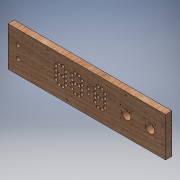
# Autodesk Inventor part: licht_200_top_b
Saved by Autodesk Inventor 2016 SP2 (Build 200236200, 236)
## iProperties
Created: 2018-01-11
Part Number: licht_200_top_b
Material: Spanplatte
Document SubType Name: Blech
Designer: schueler
Density: 1 g/cm^3
Sheet Metal Rule: Standard_mm
Appearance: Birke - natur- poliert
Mass: 590.035 g
Surface Area: 1129.46 cm^2
Volume: 590.035 cm^3
Author: schueler
Autodesk Inventor part; units mm, degrees
ref_plane "YZ Plane" through (0, 0, 0) normal (1, 0, 0) x (0, 1, 0)
ref_plane "XZ Plane" through (0, 0, 0) normal (0, 1, 0) x (-1, 0, 0)
ref_plane "XY Plane" through (0, 0, 0) normal (0, 0, 1) x (1, 0, 0)
sketch "Skizze1" plane through (0, 0, 0) normal (0, 1, 0) x (-1, 0, 0)
  line L0 (0, 0) -> (400, 0)
  line L1 (400, -100) -> (0, -100)
  line L2 (0, -100) -> (0, 0)
  line L3 (100, 0) -> (100, -100) construction
  line L4 (0, -92) -> (400, -92) construction
  circle A0 centre (100, -8) radius 1.5
  line L5 (8, 0) -> (8, -100) construction
  circle A1 centre (8, -30) radius 1.5
  circle A2 centre (8, -70) radius 1.5
  line L6 (400, -8) -> (0, -8) construction
  circle A3 centre (250, -92) radius 1.5
  line L7 (300, 0) -> (300, -100) construction
  circle A4 centre (300, -8) radius 1.5
  line L8 (400, -100) -> (400, 0)
  line L9 (250, -8) -> (250, -92) construction
  point P0 (100, -92)
  point P1 (100, -8)
  point P2 (300, -92)
  dimension "d2" = 400
  dimension "d7" = 100
  dimension "d16" = 3
  dimension "d19" = 8
  dimension "d23" = 3
  dimension "d24" = 3
  dimension "d46" = 30
  dimension "d47" = 30
  dimension "d57" = 8
  dimension "d58" = 3
  dimension "d63" = 200
  dimension "d69" = 3
  dimension "d116" = 250
  dimension "d127" = 100
  dimension "d128" = 8
  constraints: 22 point on line, 21 end point, 5 centre point, 5 perpendicular, 1 coincident, 1 horizontal, 1 parallel, 1 vertical
  measures "d2" distance of L1.start L1.end
  measures "d7" distance of L0.start L3.start
  measures "d16" diameter of A0
  measures "d19" distance of L0.start L5.start
  measures "d23" diameter of A1
  measures "d24" diameter of A2
  measures "d46" distance from line of L0 A1.centre
  measures "d47" distance from line of L1 A2.centre
  measures "d57" distance between parallel lines of L0 L6
  measures "d58" diameter of A3
  measures "d63" distance between parallel lines of L3 L7
  measures "d69" diameter of A4
  measures "d116" distance from line of L2 L9.start
  measures "d127" distance between parallel lines of L0 L1
  measures "d128" distance between parallel lines of L1 L4
extrude "Extrusion9" add sketch "Skizze1" along normal blind 16
sketch "Skizze6" plane through (0, 0, 0) normal (0, -1, 0) x (1, 0, 0)
  line L0 (-400, -100) -> (0, -100) construction
  line L1 (0, -100) -> (0, 0) construction
  line L2 (0, 0) -> (-400, 0) construction
  line L3 (-400, 0) -> (-400, -100) construction
  line L4 (0, -50) -> (-400, -50) construction
  line L5 (-400, 0) -> (-400, -100) construction
  line L6 (0, 0) -> (-400, 0) construction
  line L7 (-400, -100) -> (0, -100) construction
  line L8 (-254, 0) -> (-254, -100) construction
  line L9 (-261.5, 0) -> (-261.5, -100) construction
  line L10 (-271.5, 0) -> (-271.5, -100) construction
  line L11 (-279, 0) -> (-279, -100) construction
  line L12 (-238, 0) -> (-238, -100) construction
  line L13 (-230.5, 0) -> (-230.5, -100) construction
  line L14 (-220.5, 0) -> (-220.5, -100) construction
  line L15 (-213, 0) -> (-213, -102.7121) construction
  line L16 (-179, 0) -> (-179, -100) construction
  line L17 (-171.5, 0) -> (-171.5, -100) construction
  line L18 (-161.5, 0) -> (-161.5, -100) construction
  line L19 (-154, 0) -> (-154, -100) construction
  line L20 (-279, -41.5) -> (-154, -41.5) construction
  line L21 (-154, -31.5) -> (-279, -31.5) construction
  line L22 (-279, -24) -> (-154, -24) construction
  line L23 (-279, -51.5) -> (-154, -51.5) construction
  line L24 (-154, -61.5) -> (-279, -61.5) construction
  line L25 (-279, -69) -> (-154, -69) construction
  line L26 (-250, 0) -> (-250, -100) construction
  line L27 (-196, -61.5) -> (-196, -41.5) construction
  point P0 (-271.5, -69)
  point P1 (-261.5, -69)
  point P2 (-254, -61.5)
  point P3 (-254, -51.5)
  point P4 (-271.5, -24)
  point P5 (-261.5, -24)
  point P6 (-254, -31.5)
  point P7 (-254, -41.5)
  point P8 (-238, -41.5)
  point P9 (-238, -31.5)
  point P10 (-230.5, -24)
  point P11 (-220.5, -24)
  point P12 (-213, -31.5)
  point P13 (-213, -41.5)
  point P14 (-238, -51.5)
  point P15 (-238, -61.5)
  point P16 (-230.5, -69)
  point P17 (-220.5, -69)
  point P18 (-213, -61.5)
  point P19 (-213, -51.5)
  point P20 (-171.5, -24)
  point P21 (-161.5, -24)
  point P22 (-179, -31.5)
  point P23 (-179, -41.5)
  point P24 (-161.5, -69)
  point P25 (-171.5, -69)
  point P26 (-179, -61.5)
  point P27 (-179, -51.5)
  point P28 (-375, -35)
  point P29 (-375, -65)
  point P30 (-196, -52)
  point P31 (-196, -41)
  point P32 (-271.5, -46.5)
  point P33 (-261.5, -46.5)
  point P34 (-230.5, -46.5)
  point P35 (-220.5, -46.5)
  point P36 (-171.5, -46.5)
  point P37 (-161.5, -46.5)
  dimension "d137" = 7.5
  dimension "d139" = 7.5
  dimension "d141" = 7.5
  dimension "d143" = 7.5
  dimension "d145" = 7.5
  dimension "d147" = 7.5
  dimension "d149" = 10
  dimension "d150" = 7.5
  dimension "d152" = 10
  dimension "d153" = 7.5
  dimension "d201" = 17
  dimension "d215" = 25
  dimension "d216" = 66
  dimension "d217" = 25
  dimension "d218" = 25
  dimension "d220" = 17
  dimension "d221" = 154
  dimension "d222" = 45
  dimension "d223" = 24
  dimension "d224" = 15
  dimension "d225" = 15
  dimension "d226" = 25
  dimension "d228" = 11
  dimension "d229" = 10
  dimension "d230" = 5
  dimension "d232" = 48
  constraints: 78 point on line, 50 end point, 12 perpendicular, 8 coincident, 8 parallel, 5 horizontal alignment, 3 vertical, 2 midpoint, 1 horizontal, 1 vertical alignment, 27 other
  measures "d137" distance between parallel lines of L12 L13
  measures "d139" distance between parallel lines of L15 L14
  measures "d141" distance between parallel lines of L9 L8
  measures "d143" distance between parallel lines of L10 L11
  measures "d145" distance between parallel lines of L17 L16
  measures "d147" distance between parallel lines of L19 L18
  measures "d149" distance between parallel lines of L20 L21
  measures "d150" distance between parallel lines of L21 L22
  measures "d152" distance between parallel lines of L23 L24
  measures "d153" distance between parallel lines of L24 L25
  measures "d201" distance between parallel lines of L15 L27
  measures "d215" distance between parallel lines of L19 L16
  measures "d216" distance between parallel lines of L11 L15
  measures "d217" distance between parallel lines of L11 L8
  measures "d218" distance between parallel lines of L12 L15
  measures "d220" distance between parallel lines of L16 L27
  measures "d221" distance between parallel lines of L19 L1
  measures "d222" distance between parallel lines of L25 L22
  measures "d223" distance between parallel lines of L2 L22
  measures "d224" distance from line of point (-375, -35) L4
  measures "d225" distance from line of L4 point (-375, -65)
  measures "d226" distance from line of L3 point (-375, -65)
  measures "d228" distance of point (-196, -41) point (-196, -52)
  measures "d229" distance of L23.start point (-279, -41.5)
  measures "d230" distance from line of point (-271.5, -46.5) L20
hole "Bohrung5" at (-271.5, 0, -69) at (-261.5, 0, -69) at (-254, 0, -61.5) at (-254, 0, -51.5) at (-279, 0, -51.5) at (-279, 0, -61.5) at (-279, 0, -41.5) at (-279, 0, -31.5) at (-271.5, 0, -24) at (-261.5, 0, -24) at (-254, 0, -31.5) at (-254, 0, -41.5) at (-238, 0, -41.5) at (-238, 0, -31.5) at (-230.5, 0, -24) at (-220.5, 0, -24) at (-213, 0, -31.5) at (-213, 0, -41.5) at (-238, 0, -51.5) at (-238, 0, -61.5) at (-230.5, 0, -69) at (-220.5, 0, -69) at (-213, 0, -61.5) at (-213, 0, -51.5) at (-171.5, 0, -24) at (-161.5, 0, -24) at (-179, 0, -31.5) at (-179, 0, -41.5) at (-154, 0, -51.5) at (-154, 0, -61.5) at (-161.5, 0, -69) at (-171.5, 0, -69) at (-179, 0, -61.5) at (-179, 0, -51.5) at (-154, 0, -41.5) at (-154, 0, -31.5) at (-196, 0, -41) at (-196, 0, -52) at (-271.5, 0, -46.5) at (-261.5, 0, -46.5) at (-230.5, 0, -46.5) at (-220.5, 0, -46.5) at (-171.5, 0, -46.5) at (-161.5, 0, -46.5) direction (0, 1, 0) diameter 6 depth 30 tip angle 118 counterbore diameter 8 counterbore depth 12
hole "Bohrung6" at (-375, 0, -35) at (-375, 0, -65) direction (0, 1, 0) diameter 7 depth 30 tip angle 118 counterbore diameter 10 counterbore depth 12
sketch "Skizze7" plane through (0, 16, 0) normal (0, 1, 0) x (1, 0, 0)
  circle A0 centre (-250, 92) radius 1.5 projected
  circle A1 centre (-300, 8) radius 1.5 projected
  circle A2 centre (-8, 70) radius 1.5 projected
  circle A3 centre (-8, 30) radius 1.5 projected
  circle A4 centre (-100, 8) radius 1.5 projected
  line L0 (0, 0) -> (-400, 0) construction
  line L1 (-400, 0) -> (-400, 100) construction
  line L2 (-400, 100) -> (0, 100) construction
  line L3 (0, 100) -> (0, 0) construction
  line L4 (-40, 50) -> (0, 50) construction
  line L5 (0, 0) -> (0, 100) construction
  line L6 (-25.4, 35.4) -> (-54.6, 35.4) construction
  line L7 (-54.6, 35.4) -> (-54.6, 64.6) construction
  line L8 (-54.6, 64.6) -> (-25.4, 64.6) construction
  line L9 (-25.4, 64.6) -> (-25.4, 35.4) construction
  line L10 (-40, 50) -> (-40, 100) construction
  circle A5 centre (-40, 50) radius 25.4 construction
  line L11 (-100, 0) -> (-100, 100) construction
  line L12 (-85.4, 35.4) -> (-114.6, 35.4) construction
  line L13 (-114.6, 35.4) -> (-114.6, 64.6) construction
  line L14 (-114.6, 64.6) -> (-85.4, 64.6) construction
  line L15 (-85.4, 64.6) -> (-85.4, 35.4) construction
  circle A6 centre (-100, 50) radius 25.4 construction
  point P0 (-54.6, 50)
  point P1 (-40, 64.6)
  point P2 (-100, 35.4)
  dimension "d184" = 40
  dimension "d185" = 29.2
  dimension "d186" = 29.2
  dimension "d202" = 50.8
  dimension "d203" = 60
  dimension "d204" = 29.2
  dimension "d205" = 29.2
  dimension "d206" = 50.8
  constraints: 30 end point, 10 coincident, 6 parallel, 6 perpendicular, 6 point on line, 5 midpoint, 3 horizontal, 2 centre point, 1 collinear
  measures "d184" distance between parallel lines of L3 L10
  measures "d185" distance of L6.start L6.end
  measures "d186" distance between parallel lines of L8 L6
  measures "d202" diameter of A5
  measures "d203" distance between parallel lines of L11 L10
  measures "d204" distance of L12.start L12.end
  measures "d205" distance of L12.end L13.end
  measures "d206" diameter of A6
hole "Bohrung7" at (-100, 16, -8) at (-250, 16, -92) at (-300, 16, -8) at (-8, 16, -70) at (-8, 16, -30) direction (0, -1, 0) diameter 4 end through all countersink diameter 8 countersink angle 90
hole "Bohrung8" at (-40, 16, -50) at (-100, 16, -50) direction (0, -1, 0) diameter 24 end through all
hole "Bohrung9" at (-54.6, 16, -64.6) at (-25.4, 16, -35.4) at (-25.4, 16, -64.6) at (-54.6, 16, -35.4) at (-85.4, 16, -35.4) at (-85.4, 16, -64.6) at (-114.6, 16, -64.6) at (-114.6, 16, -35.4) direction (0, -1, 0) diameter 1.5 end through all
sketch "Skizze9" plane through (0, 16, 0) normal (0, 1, 0) x (1, 0, 0)
  circle A0 centre (-100, 50) radius 12 projected
  line L0 (-82.5, 42.5) -> (-117.5, 42.5)
  line L1 (-117.5, 42.5) -> (-117.5, 57.5)
  line L2 (-117.5, 57.5) -> (-82.5, 57.5)
  line L3 (-82.5, 57.5) -> (-82.5, 42.5)
  line L4 (-100, 50) -> (-100, 42.5) construction
  line L5 (-100, 50) -> (-117.5, 50) construction
  point P0 (0, 0)
  dimension "d211" = 15
  dimension "d212" = 35
  constraints: 12 end point, 2 midpoint, 2 parallel, 2 perpendicular, 1 horizontal, 1 vertical
  measures "d211" distance of L0.end L1.end
  measures "d212" distance of L0.start L0.end
extrude "Extrusion11" cut sketch "Skizze9" against normal blind 2 contours A0 L0 L2 | A0 L2 L3 L0 | A0 L0 L1 L2
equation "\"Biegeradius\" = Stärke"
equation "\"BreiteBiegungsfreistellung\" = Stärke"
equation "\"TiefeBiegungsfreistellung\" = 0.5 * Stärke"
equation "\"GrößeEckenfreistellung\" = 4 * Stärke"
equation "\"MinimalRest\" = 2 * Stärke"
equation "\"Übergangsradius\" = Biegeradius"
equation "\"JacobiRadiusGröße\" = Biegeradius"
equation "\"Abstandsgröße\" = Stärke"
equation "\"Stärke\" = 0.5"
